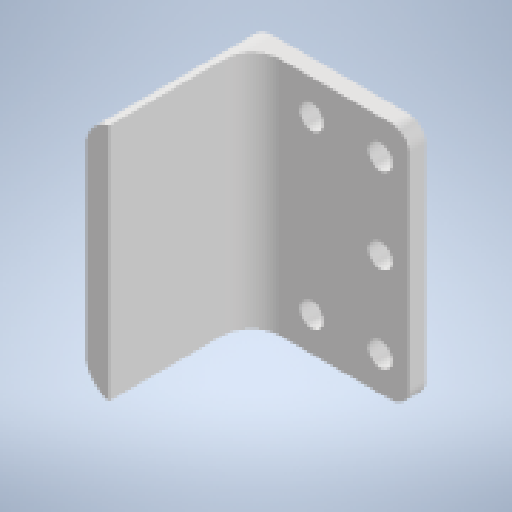
# Autodesk Inventor part: 拖带架
Saved by Autodesk Inventor 2025.1 (Build 291241000, 241)
## iProperties
Created: 2025-08-31
Part Number: 拖带架
Material: 常规
Document SubType Name: Modeling
Designer: Piw
Density: 1 g/cm^3
Appearance: 默认
Author: Piw
Autodesk Inventor part; units mm, degrees
ref_plane "YZ Plane" through (0, 0, 0) normal (1, 0, 0) x (0, 1, 0)
ref_plane "XZ Plane" through (0, 0, 0) normal (0, 1, 0) x (-1, 0, 0)
ref_plane "XY Plane" through (0, 0, 0) normal (0, 0, 1) x (1, 0, 0)
sketch "草图2" plane through (0, 0, 0) normal (0, 0, 1) x (1, 0, 0)
  circle A0 centre (8, 60) radius 2.1 projected
  circle A1 centre (20, 60) radius 2.1 projected
  circle A2 centre (20, 75) radius 2.1 projected
  circle A3 centre (20, 90) radius 1.75 projected
  circle A4 centre (8, 90) radius 2.1 projected
  line L0 (22, 54) -> (0, 54) projected
  arc A5 (22, 54) -> (25, 57) centre (22, 57) ccw projected
  line L1 (25, 93) -> (25, 57) projected
  line L2 (0, 96) -> (22, 96) projected
  arc A6 (25, 93) -> (22, 96) centre (22, 93) ccw projected
  line L3 (0, 96) -> (-6.5, 96)
  line L4 (-6.5, 96) -> (-6.5, 54)
  line L5 (-6.5, 54) -> (0, 54)
  line L6 (0, 54) -> (0, 96)
  circle A7 centre (20, 60) radius 2.1
  circle A8 centre (8, 60) radius 2.1
  circle A9 centre (20, 75) radius 2.1
  circle A10 centre (20, 90) radius 2.1
  circle A11 centre (8, 90) radius 2.1
  point P0 (0, 0)
  dimension "d0" = 6.5
  dimension "d11" = 4.2
  dimension "d12" = 4.2
  dimension "d13" = 4.2
  dimension "d14" = 4.2
  dimension "d15" = 4.2
  constraints: 8 end point, 5 centre point, 5 coincident, 2 parallel, 1 collinear, 1 horizontal, 1 perpendicular
  measures "d0" distance of L4.end L5.end
  measures "d11" diameter of A7
  measures "d12" diameter of A8
  measures "d13" diameter of A9
  measures "d14" diameter of A10
  measures "d15" diameter of A11
extrude "拉伸1" add sketch "草图2" along normal blind 3 contours L0 L6 L2 A6 L1 A5 | L5 L4 L3 L6
sketch "草图3" plane through (0, 0, 3) normal (0, 0, 1) x (1, 0, 0)
  line L0 (-6.5, 54) -> (22, 54) projected
  line L1 (22, 96) -> (-6.5, 96) projected
  line L2 (-6.5, 54) -> (-2.5, 54)
  line L3 (-2.5, 54) -> (-2.5, 96)
  line L4 (-2.5, 96) -> (-6.5, 96)
  line L5 (-6.5, 96) -> (-6.5, 54)
  point P0 (0, 0)
  dimension "d3" = 4
  constraints: 8 end point, 2 parallel, 1 horizontal, 1 perpendicular, 1 point on line
  measures "d3" distance between parallel lines of L5 L3
extrude "拉伸2" add sketch "草图3" along normal blind 25
fillet "圆角1" radius 5 1 edges at (-2.5, 75, 3)
fillet "圆角2" radius 5 2 edges at (-6.5, 96, 14) (-6.5, 54, 14)
